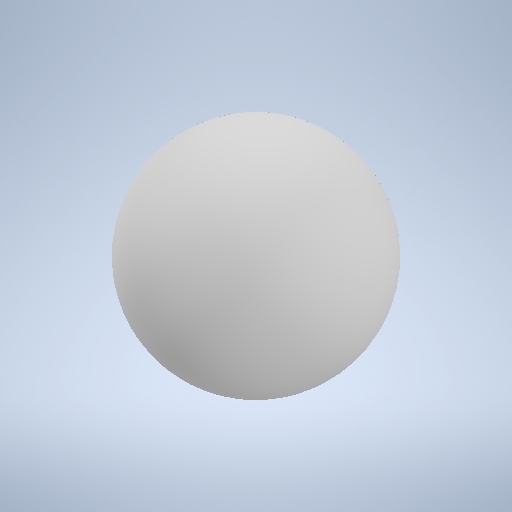
# Autodesk Inventor part: Part1
Saved by Autodesk Inventor 2025.4 (Build 294407000, 407)
## iProperties
Created: 2026-03-03
Part Number: Part1
Material: Generic
Document SubType Name: Modeling
Designer: Amir
Density: 1 g/cm^3
Appearance: Default
Author: Amir
Autodesk Inventor part; units mm, degrees
ref_plane "YZ Plane" through (0, 0, 0) normal (1, 0, 0) x (0, 1, 0)
ref_plane "XZ Plane" through (0, 0, 0) normal (0, 1, 0) x (-1, 0, 0)
ref_plane "XY Plane" through (0, 0, 0) normal (0, 0, 1) x (1, 0, 0)
sketch "Sketch1" plane through (0, 0, 0) normal (0, 0, 1) x (1, 0, 0)
  arc A0 (15, 0) -> (-15, 0) centre (0, 0) ccw
  arc A1 (12.5, 0) -> (-12.5, 0) centre (0, 0) ccw
  line L0 (-18.0373, 0) -> (31.5731, 0)
  dimension "d0" = 30
  dimension "d1" = 25
  constraints: 4 point on circle, 4 point on line, 2 centre point, 2 coincident, 2 end point, 1 horizontal
  measures "d0" diameter of A0
  measures "d1" diameter of A1
revolve "Revolution1" add sketch "Sketch1" angle 360 about axis through (-18.0373, 0, 0) along (1, 0, 0) contours L0 A1 A0
body "Solid1"
